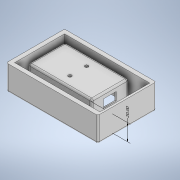
# Autodesk Inventor part: abajo model2
Saved by Autodesk Inventor 2020 (Build 240168000, 168)
## iProperties
Created: 2022-05-31
Part Number: abajo model2
Material: Generic
Document SubType Name: Modeling
Designer: juanc
Density: 1 g/cm^3
Appearance: Default
Author: juanc
Autodesk Inventor part; units mm, degrees
ref_plane "YZ Plane" through (0, 0, 0) normal (1, 0, 0) x (0, 1, 0)
ref_plane "XZ Plane" through (0, 0, 0) normal (0, 1, 0) x (-1, 0, 0)
ref_plane "XY Plane" through (0, 0, 0) normal (0, 0, 1) x (1, 0, 0)
sketch "Sketch1" plane through (0, 0, 0) normal (0, 1, 0) x (-1, 0, 0)
  line L0 (0, 0) -> (100, 0)
  line L1 (100, 0) -> (100, -60)
  line L2 (100, -60) -> (0, -60)
  line L3 (0, -60) -> (0, 0)
  line L4 (100, -52.4106) -> (95, -52.4106) construction
  line L5 (100, -52.4106) -> (105, -52.4106) construction
  line L6 (95, -60) -> (95, -55)
  line L7 (95, -55) -> (22, -55)
  line L8 (22, -55) -> (22, -15)
  line L9 (22, -15) -> (95, -15)
  line L10 (95, -15) -> (95, -55)
  line L11 (100, 0) -> (0, -60) construction
  line L12 (100, -60) -> (0, 0) construction
  line L13 (-5, -65) -> (105, -65)
  line L14 (105, -65) -> (105, 5)
  line L15 (105, 5) -> (-5, 5)
  line L16 (-5, 5) -> (-5, -65)
  line L17 (-5, -65) -> (105, 5) construction
  line L18 (105, -65) -> (-5, 5) construction
  line L19 (95, -15) -> (22, -55) construction
  line L20 (95, -55) -> (22, -15) construction
  line L21 (20.5, -13) -> (96.5, -13)
  line L22 (96.5, -13) -> (96.5, -57)
  line L23 (96.5, -57) -> (20.5, -57)
  line L24 (20.5, -57) -> (20.5, -13)
  line L25 (20.5, -13) -> (96.5, -57) construction
  line L26 (96.5, -13) -> (20.5, -57) construction
  point P0 (50, -30)
  point P1 (58.5, -35)
  dimension "d0" = 100
  dimension "d1" = 60
  dimension "d2" = 5
  dimension "d3" = 180
  dimension "d4" = 5
  dimension "d5" = 73
  dimension "d6" = 40
  dimension "d7" = 110
  dimension "d8" = 70
  dimension "d9" = 76
  dimension "d10" = 44
  constraints: 54 end point, 8 parallel, 6 horizontal, 6 midpoint, 5 perpendicular, 2 point on line, 1 collinear
  measures "d0" distance of L1.end L2.end
  measures "d1" distance of L0.end L1.end
  measures "d2" distance of L4.start L4.end
  measures "d3" angle of L4 L5
  measures "d4" distance of L6.start L6.end
  measures "d5" distance of L8.end L9.end
  measures "d6" distance of L7.end L8.end
  measures "d7" distance of L15.end L14.end
  measures "d8" distance of L14.end L13.end
  measures "d9" distance of L22.end L23.end
  measures "d10" distance of L21.end L22.end
extrude "Extrusion1" add sketch "Sketch1" along normal blind 30 contours L16 L15 L14 L13
extrude "Extrusion2" add sketch "Sketch1" along normal blind 22 contours L21 L22 L23 L24
extrude "Extrusion3" add sketch "Sketch1" along normal blind 2.5 contours L0 L1 L2 L3
sketch "Sketch2" plane through (0, 22, 0) normal (0, 1, 0) x (1, 0, 0)
  line L0 (-20.5, 57) -> (-96.5, 57) projected
  line L1 (-96.5, 13) -> (-20.5, 13) projected
  line L2 (-96.5, 57) -> (-20.5, 57)
  line L3 (-20.5, 57) -> (-20.5, 13)
  line L4 (-20.5, 13) -> (-96.5, 13)
  line L5 (-96.5, 13) -> (-96.5, 57)
  point P0 (0, 0)
  constraints: 8 end point, 2 parallel, 1 horizontal, 1 perpendicular
extrude "Extrusion4" add sketch "Sketch2" along normal blind 2.5
sketch "Sketch4" plane through (-20.5, 2.5, -13) normal (1, 0, 0) x (0, 0, -1)
  line L0 (-18, -2.5) -> (-18, 27.5) projected
  line L1 (-18, 27.5) -> (-13, 27.5) projected
  line L2 (-13, 27.5) -> (-13, 0) projected
  line L3 (-13, 0) -> (0, 0) projected
  line L4 (0, 0) -> (44, 0) projected
  line L5 (44, 0) -> (47, 0) projected
  line L6 (47, 0) -> (47, 27.5) projected
  line L7 (47, 27.5) -> (52, 27.5) projected
  line L8 (52, 27.5) -> (52, -2.5) projected
  line L9 (52, -2.5) -> (-18, -2.5) projected
  line L10 (0, 0) -> (0, 22) projected
  line L11 (0, 22) -> (44, 22) projected
  line L12 (44, 22) -> (44, 0) projected
  line L13 (0, 22) -> (44, 22) projected
  line L14 (44, 22) -> (0, 22) projected
  line L15 (-18, -2.5) -> (52, -2.5) projected
  line L16 (52, -2.5) -> (52, 27.5) projected
  line L17 (-18, 27.5) -> (52, 27.5) projected
  line L18 (-18, -2.5) -> (-18, 27.5) projected
  line L19 (0, 0) -> (44, 0) projected
  line L20 (44, 0) -> (44, 22) projected
  line L21 (0, 22) -> (44, 22) projected
  line L22 (0, 0) -> (0, 22) projected
  line L23 (44, 0) -> (44, 22) construction
  line L24 (44, 22) -> (0, 0) construction
  line L25 (44, 0) -> (0, 0) construction
  line L26 (44, 22) -> (0, 22) construction
  line L27 (44, 0) -> (0, 22) construction
  line L28 (29.5, 6) -> (14.5, 6)
  line L29 (14.5, 6) -> (14.5, 16)
  line L30 (14.5, 16) -> (29.5, 16)
  line L31 (29.5, 16) -> (29.5, 6)
  line L32 (29.5, 6) -> (14.5, 16) construction
  line L33 (14.5, 6) -> (29.5, 16) construction
  point P0 (-13, -2.5)
  point P1 (22, 11)
  dimension "d19" = 15
  dimension "d20" = 10
  constraints: 16 end point, 3 midpoint, 2 parallel, 1 horizontal, 1 perpendicular
  measures "d19" distance of L29.end L30.end
  measures "d20" distance of L28.end L29.end
extrude "Extrusion5" cut sketch "Sketch4" against normal blind 10 contours L28 L29 L30 L31
fillet "Fillet1" radius 2 8 edges at (-58.5, 24.5, -57) (-20.5, 24.5, -35) (-58.5, 24.5, -13) (-96.5, 24.5, -35) (-20.5, 13.5, -13) (-20.5, 13.5, -57) (-96.5, 13.5, -13) (-96.5, 13.5, -57)
sketch "Sketch5" plane through (0, 22, 0) normal (0, -1, 0) x (1, 0, 0)
  line L0 (-22, -55) -> (-22, -15) construction
  line L1 (-94.5, -55) -> (-96.5, -55) construction
  line L2 (-58.5, -35) -> (-58.5, -55) construction
  line L3 (-58.5, -55) -> (-58.5, -45) construction
  line L4 (-58.5, -15) -> (-58.5, -25) construction
  point P0 (0, 0)
  dimension "d24" = 10
  dimension "d25" = 10
  constraints: 6 end point, 2 coincident, 2 vertical, 1 midpoint
  measures "d24" distance of L2.end L3.end
  measures "d25" distance of L4.start L4.end
hole "Hole1" at (-58.5, 22, -45) at (-58.5, 22, -25) direction (0, 1, 0) diameter 1.5 depth 40 tip angle 118
sketch "Sketch6" plane through (0, 24.5, 0) normal (0, 1, 0) x (1, 0, 0)
  circle A0 centre (-58.5, 45) radius 0.75 projected
  circle A1 centre (-58.5, 45) radius 2
  circle A2 centre (-58.5, 25) radius 0.75 projected
  circle A3 centre (-58.5, 25) radius 2
  point P0 (0, 0)
  dimension "d33" = 4
  dimension "d34" = 4
  constraints: 2 centre point, 2 coincident
  measures "d33" diameter of A1
  measures "d34" diameter of A3
extrude "Extrusion6" cut sketch "Sketch6" against normal blind 1.5
fillet "Fillet2" radius 2 4 edges at (-50, 0, -65) (-105, 0, -30) (-50, 0, 5) (5, 0, -30)
sketch "Sketch7" plane through (0, 30, 0) normal (0, 1, 0) x (1, 0, 0)
  line L0 (0, 60) -> (2.5, 60)
  line L1 (2.5, 60) -> (2.5, 0)
  line L2 (2.5, 0) -> (0, 0)
  line L3 (0, 0) -> (0, 60)
  dimension "d46" = 2.5
  constraints: 8 end point, 2 parallel, 1 horizontal, 1 perpendicular
  measures "d46" distance of L1.end L2.end
extrude "Extrusion7" cut sketch "Sketch7" against normal blind 27.5
fillet "Fillet3" radius 2 8 edges at (-104.4142, 0.5858, 4.4142) (-105, 16, 5) (4.4142, 0.5858, 4.4142) (5, 16, 5) (-104.4142, 0.5858, -64.4142) (-105, 16, -65) (4.4142, 0.5858, -64.4142) (5, 16, -65)
body "Solid1"
